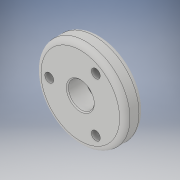
# Autodesk Inventor part: Piston of Suspension
Saved by Autodesk Inventor 2019 (Build 230136000, 136)
## iProperties
Created: 2019-11-29
Part Number: Piston of Suspension
Material: Generic
Document SubType Name: Modeling
Designer: Jopa
Density: 1 g/cm^3
Appearance: Default
Author: Jopa
Autodesk Inventor part; units mm, degrees
ref_plane "YZ Plane" through (0, 0, 0) normal (1, 0, 0) x (0, 1, 0)
ref_plane "XZ Plane" through (0, 0, 0) normal (0, 1, 0) x (-1, 0, 0)
ref_plane "XY Plane" through (0, 0, 0) normal (0, 0, 1) x (1, 0, 0)
sketch "Sketch1" plane through (0, 0, 0) normal (0, 0, 1) x (1, 0, 0)
  circle A0 centre (0, 0) radius 1.5875
  circle A1 centre (0, 0) radius 5.461
  dimension "d0" = 3.175
  dimension "d1" = 10.922
  constraints: 2 centre point, 2 coincident
  measures "d0" diameter of A0
  measures "d1" diameter of A1
extrude "Extrusion1" add sketch "Sketch1" along normal mid plane 2.3813
fillet "Fillet1" radius 0.635 2 edges at (-5.461, 0, 1.1906) (-5.461, 0, -1.1906)
chamfer "Chamfer1" distance 0.127 angle 45 2 edges at (-1.5875, 0, 1.1906) (-1.5875, 0, -1.1906)
sketch "Sketch2" plane through (0, 0, 1.1906) normal (0, 0, 1) x (1, 0, 0)
  circle A0 centre (-3.81, 0) radius 0.5461
  point P0 (0, 0)
  dimension "d8" = 1.0922
  dimension "d9" = 3.81
  constraints: 1 centre point, 1 horizontal alignment
  measures "d8" diameter of A0
  measures "d9" distance of point (0, 0) A0.centre
extrude "Extrusion2" cut sketch "Sketch2" along normal through all both and the other way through all
pattern_circular "Circular Pattern1" count 3 over 360 about axis through (0, 0, -10) along (0, 0, 1) of "Extrusion2"
body "Solid1"
